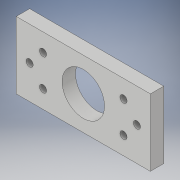
# Autodesk Inventor part: nhk45
Saved by Autodesk Inventor 2019 (Build 230136000, 136)
## iProperties
Created: 2022-02-27
Part Number: nhk45
Material: 一般
Document SubType Name: Sheet Metal
Designer: yuta
Density: 1 g/cm^3
Sheet Metal Rule: Default_mm
Appearance: 既定
Author: yuta
Autodesk Inventor part; units mm, degrees
ref_plane "YZ Plane" through (0, 0, 0) normal (1, 0, 0) x (0, 1, 0)
ref_plane "XZ Plane" through (0, 0, 0) normal (0, 1, 0) x (-1, 0, 0)
ref_plane "XY Plane" through (0, 0, 0) normal (0, 0, 1) x (1, 0, 0)
sketch "スケッチ1" plane through (0, 0, 0) normal (0, 0, 1) x (1, 0, 0)
  line L0 (0, 0) -> (60, 0)
  line L1 (60, 0) -> (60, 30)
  line L2 (60, 30) -> (0, 30)
  line L3 (0, 30) -> (0, 0)
  dimension "d0" = 60
  dimension "d1" = 30
  constraints: 8 end point, 2 parallel, 1 horizontal, 1 perpendicular
  measures "d0" distance of L2.end L1.end
  measures "d1" distance of L1.end L0.end
extrude "押し出し1" add sketch "スケッチ1" along normal blind 6
sketch "スケッチ2" plane through (0, 0, 6) normal (0, 0, 1) x (1, 0, 0)
  circle A0 centre (30, 15) radius 9.5
  line L0 (0, 30) -> (0, 0) projected
  line L1 (60, 30) -> (0, 30) projected
  dimension "d4" = 19
  dimension "d5" = 30
  dimension "d6" = 15
  constraints: 1 centre point
  measures "d4" diameter of A0
  measures "d5" distance from line of L0 A0.centre
  measures "d6" distance from line of L1 A0.centre
extrude "押し出し2" cut sketch "スケッチ2" against normal blind 6
sketch "スケッチ3" plane through (0, 0, 6) normal (0, 0, 1) x (1, 0, 0)
  circle A0 centre (12, 22) radius 1.6
  circle A1 centre (12, 8) radius 1.6
  line L0 (60, 30) -> (0, 30) projected
  line L1 (0, 0) -> (60, 0) projected
  line L2 (0, 30) -> (0, 0) projected
  circle A2 centre (6, 15) radius 1.6
  line L3 (30, 30) -> (30, 0) construction
  line L4 (0, 0) -> (60, 0) projected
  circle A3 centre (48, 22) radius 1.6
  circle A4 centre (48, 8) radius 1.6
  circle A5 centre (54, 15) radius 1.6
  dimension "d9" = 3.2
  dimension "d10" = 3.2
  dimension "d11" = 8
  dimension "d12" = 8
  dimension "d13" = 12
  dimension "d14" = 12
  dimension "d15" = 3.2
  dimension "d16" = 15
  dimension "d17" = 6
  constraints: 6 centre point, 3 symmetric about line, 2 end point, 2 midpoint, 3 other
  measures "d9" diameter of A0
  measures "d10" diameter of A1
  measures "d11" distance from line of L0 A0.centre
  measures "d12" distance from line of L1 A1.centre
  measures "d13" distance from line of A0.centre L2
  measures "d14" distance from line of L2 A1.centre
  measures "d15" diameter of A2
  measures "d16" distance from line of L1 A2.centre
  measures "d17" distance from line of L2 A2.centre
hole "穴1" at (12, 22, 6) at (6, 15, 6) at (12, 8, 6) at (48, 22, 6) at (54, 15, 6) at (48, 8, 6) direction (0, 0, -1) diameter 3.2 depth 6
equation "\"BendRadius\" = Thickness"
equation "\"BendReliefWidth\" = Thickness"
equation "\"BendReliefDepth\" = 0.5 * Thickness"
equation "\"CornerReliefSize\" = 4 * Thickness"
equation "\"MinimumRemnant\" = 2 * Thickness"
equation "\"TransitionRadius\" = BendRadius"
equation "\"JacobiRadiusSize\" = BendRadius"
equation "\"GapSize\" = Thickness"
equation "\"Thickness\" = 0.5"
